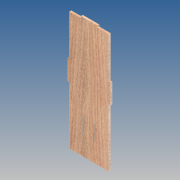
# Autodesk Inventor part: 2201_Housing Bottom_V1
Saved by Autodesk Inventor 2020 (Build 240168000, 168)
## iProperties
Created: 2019-11-08
Part Number: 2201_Housing Bottom_V1
Material: Wood (Birch)
Document SubType Name: Modeling
Designer: RFLab
Density: 0.55 g/cm^3
Appearance: Birch - Natural Polished
Author: RFLab
Autodesk Inventor part; units mm, degrees
ref_plane "YZ Plane" through (0, 0, 0) normal (1, 0, 0) x (0, 1, 0)
ref_plane "XZ Plane" through (0, 0, 0) normal (0, 1, 0) x (-1, 0, 0)
ref_plane "XY Plane" through (0, 0, 0) normal (0, 0, 1) x (1, 0, 0)
sketch "Sketch1" plane through (0, 0, 0) normal (0, 0, 1) x (1, 0, 0)
  line L0 (-75, 93.8197) -> (75, 93.8197)
  line L1 (75, 93.8197) -> (75, -336.1803)
  line L2 (75, -336.1803) -> (-75, -336.1803)
  line L3 (-75, -336.1803) -> (-75, 93.8197)
  point P0 (0, 0)
  dimension "d0" = 150
  dimension "d1" = 430
  constraints: 8 end point, 2 parallel, 1 horizontal, 1 perpendicular
  measures "d0" distance of L0.start L0.end
  measures "d1" distance of L0.end L1.end
extrude "Extrusion1" add sketch "Sketch1" along normal blind 6.35
sketch "Sketch2" plane through (0, 0, 6.35) normal (0, 0, 1) x (1, 0, 0)
  line L0 (75, 93.8197) -> (-75, 93.8197) projected
  line L1 (-75, 93.8197) -> (-68.65, 93.8197)
  line L2 (-68.65, 93.8197) -> (-68.65, -56.1803)
  line L3 (-68.65, -56.1803) -> (-75, -56.1803)
  line L4 (-75, -56.1803) -> (-75, 93.8197)
  line L5 (-75, 93.8197) -> (-75, -336.1803) projected
  line L6 (-75, -126.1803) -> (-68.65, -126.1803)
  line L7 (-68.65, -126.1803) -> (-68.65, -236.1803)
  line L8 (-68.65, -236.1803) -> (-75, -236.1803)
  line L9 (-75, -236.1803) -> (-75, -126.1803)
  line L10 (-75, 93.8197) -> (-75, -336.1803) projected
  line L11 (-75, -336.1803) -> (-68.65, -336.1803)
  line L12 (-68.65, -336.1803) -> (-68.65, -186.1803)
  line L13 (-68.65, -186.1803) -> (-75, -186.1803)
  line L14 (-75, -186.1803) -> (-75, -336.1803)
  line L15 (75, -336.1803) -> (75, 93.8197) projected
  line L16 (75, 93.8197) -> (68.65, 93.8197)
  line L17 (68.65, 93.8197) -> (68.65, -56.1803)
  line L18 (68.65, -56.1803) -> (75, -56.1803)
  line L19 (75, -56.1803) -> (75, 93.8197)
  line L20 (75, -126.1803) -> (68.65, -126.1803)
  line L21 (68.65, -126.1803) -> (68.65, -236.1803)
  line L22 (68.65, -236.1803) -> (75, -236.1803)
  line L23 (75, -236.1803) -> (75, -126.1803)
  line L24 (-75, -336.1803) -> (75, -336.1803) projected
  line L25 (75, -336.1803) -> (68.65, -336.1803)
  line L26 (68.65, -336.1803) -> (68.65, -186.1803)
  line L27 (68.65, -186.1803) -> (75, -186.1803)
  line L28 (75, -186.1803) -> (75, -336.1803)
  line L29 (-68.65, 93.8197) -> (-28.65, 93.8197)
  line L30 (-28.65, 93.8197) -> (-28.65, 87.4697)
  line L31 (-28.65, 87.4697) -> (-68.65, 87.4697)
  line L32 (-68.65, 87.4697) -> (-68.65, 93.8197)
  line L33 (68.65, 93.8197) -> (28.65, 93.8197)
  line L34 (28.65, 93.8197) -> (28.65, 87.4697)
  line L35 (28.65, 87.4697) -> (68.65, 87.4697)
  line L36 (68.65, 87.4697) -> (68.65, 93.8197)
  line L37 (-68.65, -336.1803) -> (68.9785, -336.1803)
  line L38 (68.9785, -336.1803) -> (68.9785, -329.8303)
  line L39 (-68.65, -329.8303) -> (-68.65, -336.1803)
  line L40 (68.65, -329.8303) -> (68.65, -336.1803)
  line L41 (-75, -336.1803) -> (75, -336.1803)
  line L42 (75, -336.1803) -> (75, -329.8303)
  line L43 (75, -329.8303) -> (-75, -329.8303)
  line L44 (-75, -329.8303) -> (-75, -336.1803)
  point P0 (0, 0)
  point P1 (-75, -186.1803)
  point P2 (75, -186.1803)
  point P3 (-75, -236.1803)
  point P4 (75, -236.1803)
  point P5 (75, -126.1803)
  point P6 (75, -56.1803)
  dimension "d4" = 150
  dimension "d5" = 110
  dimension "d6" = 150
  dimension "d7" = 70
  dimension "d8" = 6.35
  dimension "d9" = 6.35
  dimension "d12" = 6.35
  dimension "d13" = 6.35
  dimension "d14" = 40
  dimension "d15" = 40
  dimension "d32" = 150
  dimension "d33" = 150
  dimension "d34" = 110
  dimension "d35" = 70
  dimension "d36" = 6.35
  constraints: 80 end point, 19 parallel, 10 horizontal, 10 perpendicular, 8 point on line
  measures "d4" distance of L1.end L2.end
  measures "d5" distance of L6.end L7.end
  measures "d6" distance of L11.end L12.end
  measures "d7" distance of L6.end L2.end
  measures "d8" distance of L0.end L1.end
  measures "d9" distance of L0.start L16.end
  measures "d12" distance of L37.end L38.end
  measures "d13" distance of L29.end L30.end
  measures "d14" distance of L34.end L35.end
  measures "d15" distance of L30.end L31.end
  measures "d32" distance of L16.end L17.end
  measures "d33" distance of L25.end L26.end
  measures "d34" distance of L20.end L21.end
  measures "d35" distance of L20.end L17.end
  measures "d36" distance between parallel lines of L43 L24
extrude "Extrusion2" cut sketch "Sketch2" against normal through all contours L15 L18 L17 L0 | L17 L35 L34 L0 | L15 L27 L21 L20 | L30 L31 L2 L0 | L15 L22 L21 L27 | L2 L3 L4 L0 | L15 L43 L26 L22 | L15 L24 L38 L43 | L38 L24 L26 L43 | L26 L24 L12 L43 | L6 L7 L13 L5 | L43 L5 L8 L12 | L12 L11 L5 L43 | L13 L7 L8 L5
sketch "Sketch4" plane through (0, 0, 6.35) normal (0, 0, 1) x (1, 0, 0)
  circle A0 centre (0, -157.1803) radius 1.25
  line L0 (-68.65, -336.1803) -> (68.65, -336.1803) projected
  line L1 (28.65, 93.8197) -> (-28.65, 93.8197) projected
  circle A1 centre (0, -137.1803) radius 1.25
  line L2 (0, -207.1803) -> (20.41, -207.1803)
  circle A2 centre (20.41, -207.1803) radius 1.25
  line L3 (0, -207.1803) -> (-20.41, -207.1803)
  circle A3 centre (-20.41, -207.1803) radius 1.25
  line L4 (0, -137.1803) -> (-75, -137.1803)
  line L5 (-75, -56.1803) -> (-75, -126.1803) projected
  line L6 (-75, -137.1803) -> (-75, -126.1803)
  line L7 (0, -157.1803) -> (0, -137.1803)
  line L8 (0, -207.1803) -> (0, -157.1803)
  circle A4 centre (-20.41, -262.1803) radius 1.25
  circle A5 centre (20.41, -262.1803) radius 1.25
  line L9 (-21.66, -262.1803) -> (-21.66, -207.1803)
  line L10 (-19.16, -262.1803) -> (-19.16, -207.1803)
  line L11 (19.16, -262.1803) -> (19.16, -207.1803)
  line L12 (21.66, -207.1803) -> (21.66, -262.1803)
  line L13 (21.66, -262.1803) -> (19.16, -262.1803)
  line L14 (-75, -56.1803) -> (-75, -126.1803) projected
  point P0 (0, 0)
  point P1 (-28.65, -336.1803)
  point P2 (28.65, -336.1803)
  point P3 (-75, -236.1803)
  point P4 (-75, -306.1803)
  dimension "d18" = 2.5
  dimension "d22" = 251
  dimension "d23" = 20
  dimension "d25" = 20.41
  dimension "d26" = 75
  dimension "d27" = 50
  dimension "d28" = 55
  dimension "d30" = 55
  dimension "d31" = 55
  constraints: 22 end point, 8 point on circle, 6 centre point, 5 equal radius, 5 parallel, 3 collinear, 3 horizontal, 3 point on line, 2 coincident, 2 perpendicular, 1 tangent
  measures "d18" diameter of A0
  measures "d22" distance from line of L1 L7.start
  measures "d23" distance of L4.start L7.start
  measures "d25" distance of L2.start L2.end
  measures "d26" distance of L4.start L4.end
  measures "d27" distance of L2.start L7.start
  measures "d28" distance of L9.start L9.end
  measures "d30" distance of L11.start L11.end
  measures "d31" distance of L10.start L10.end
extrude "Extrusion3" cut sketch "Sketch4" against normal through all
equation "\"d9\" = d8"
equation "\"d13\" = d8"
equation "\"d15\" = d14"
equation "\"d32\" = d4"
equation "\"d33\" = d6"
equation "\"d34\" = d5"
equation "\"d35\" = d7"
equation "\"d30\" = d28"
body "Solid1"
